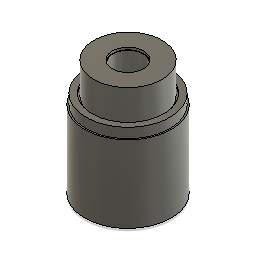
shaft (Autodesk Fusion 360 design; units mm, degrees)
Autodesk Fusion 360 part; units mm, degrees
note: some values were not read from the file. Chosen so that the rebuilt part matches the saved one: which face or edge a step refers to; where a thread starts. Set by a fixed rule: which sketch regions a step uses.
sketch "Sketch1" plane through (0, 0, 0) normal (0, 1, 0) x (1, 0, 0) in component "Eixo"
  circle A0 centre (0, 0) radius 7.5
  dimension "d1" = 15
  constraint coincident A0.centre origin
  measures "d1" diameter of A0
extrude "Extrude1" add sketch "Sketch1" along normal blind 25 in component "Eixo"
sketch "Sketch2" plane through (0, 25, 0) normal (0, 1, 0) x (-1, 0, 0) in component "Eixo"
  circle A0 centre (0, 0) radius 7.5
  circle A1 centre (0, 0) radius 5.9
  dimension "d4" = 11.8
  constraint concentric A0 A1
  measures "d4" diameter of A1
extrude "Extrude2" add sketch "Sketch2" along normal blind 5 contours A1 in component "Eixo"
sketch "Sketch3" plane through (0, 30, 0) normal (0, 1, 0) x (-1, 0, 0) in component "Eixo"
  circle A0 centre (0, 0) radius 5.9
  circle A1 centre (0, 0) radius 2.45
  dimension "d7" = 4.9
  constraint coincident A0.centre A1.centre
  measures "d7" diameter of A1
extrude "Extrude3" add sketch "Sketch3" along normal blind 16 contours A1 in component "Eixo"
sketch "Sketch5" plane through (0, 0, 0) normal (0, -1, 0) x (1, 0, 0) in component "Eixo"
  circle A0 centre (0, 0) radius 7.5
  circle A1 centre (0, 0) radius 3.965
  dimension "d13" = 7.93
  constraint coincident A0.centre A1.centre
  measures "d13" diameter of A1
extrude "Extrude5" cut sketch "Sketch5" against normal blind 20 contours A1 in component "Eixo"
thread "Thread2" "ANSI Unified Screw Threads 0.375 3/8-16 UNC 3B" major diameter 9.525 minor diameter 7.94 pitch 1.5875 angle 60 modelled right hand crest width 0.1984 on face at (3.9521, 13.3333, -0.319) crest through (3.97, -0.893, 0) in component "Eixo"
sketch "Sketch6" plane through (0, 25, 0) normal (0, 1, 0) x (-1, 0, 0) in component "Eixo"
  circle A0 centre (0, 0) radius 5.9
  circle A1 centre (0, 0) radius 7.5
  circle A2 centre (0, 0) radius 7.25
  circle A3 centre (0, 0) radius 6.2
  dimension "d16" = 14.5
  dimension "d17" = 12.4
  constraint coincident A0.centre A1.centre
  measures "d16" diameter of A2
  measures "d17" diameter of A3
extrude "Extrude6" cut sketch "Sketch6" against normal blind 0.2 contours A1 in component "Eixo"
sketch "Sketch7" plane through (0, 25, 0) normal (0, 1, 0) x (-1, 0, 0) in component "Eixo"
  circle A0 centre (0, 0) radius 7.25
  circle A1 centre (0, 0) radius 5.9
  circle A2 centre (0, 0) radius 6.2
  dimension "d20" = 12.4
  constraint coincident A0.centre A1.centre
  measures "d20" diameter of A2
extrude "Extrude7" cut sketch "Sketch7" against normal blind 0.4 contours A2 in component "Eixo"
sketch "Sketch8" plane through (0, 30, 0) normal (0, 1, 0) x (-1, 0, 0) in component "Eixo"
  circle A0 centre (0, 0) radius 2.45
  circle A1 centre (0, 0) radius 5.9
  circle A2 centre (0, 0) radius 2.7
  dimension "d23" = 5.4
  constraint coincident A0.centre A1.centre
  measures "d23" diameter of A2
extrude "Extrude8" cut sketch "Sketch8" against normal blind 0.4 contours A2 in component "Eixo"
sketch "Sketch1 (2)" plane through (0, 0, 0) normal (0, -1, 0) x (1, 0, 0)
  spline S0 degree 3 poles (1.1325, -4.6259) (0.5322, -4.7157) (-0.0797, -4.6894) (-1.2366, -4.4049) (-1.7725, -4.1576) (-2.6991, -3.4812) (-3.0858, -3.0652) (-3.6202, -2.1947) (-3.7952, -1.767) (-3.9926, -0.8864) (-4.0186, -0.4407) (-3.97, 0) knots 0 0 0 0 0.182097 0.182097 0.357707 0.357707 0.526827 0.526827 0.664894 0.664894 0.79837 0.79837 0.79837 0.79837
  arc A0 (-2.8072, 2.8072) -> (-3.97, 0) centre (0, 0) ccw
  spline S1 degree 3 poles (-2.8072, 2.8072) (-2.4792, 3.2165) (-2.073, 3.5564) (-1.1358, 4.0756) (-0.6098, 4.2428) (0.4983, 4.3727) (1.0705, 4.3259) (2.1003, 4.0381) (2.5558, 3.8234) (3.3925, 3.2469) (3.765, 2.885) (4.0718, 2.4702) knots 0 0 0 0 0.157342 0.157342 0.321158 0.321158 0.491446 0.491446 0.641085 0.641085 0.795325 0.795325 0.795325 0.795325
  arc A1 (1.1325, -4.6259) -> (4.0718, 2.4702) centre (0, 0) ccw
  circle A2 centre (0, 0) radius 7.5
  circle A3 centre (0, 0) radius 7.5
  constraint concentric A0 A3
extrude "Extrude9" cut sketch "Sketch1 (2)" against normal blind 10 contours S0 A0 S1 A1 | A2 A3 in component "Eixo"
sketch "Sketch2 (2)" plane through (0, 46, 0) normal (0, 1, 0) x (-1, 0, 0)
  circle A0 centre (0, 0) radius 2.45
  circle A1 centre (0, 0) radius 2.6
  dimension "d28" = 5.2
  constraint coincident A0.centre A1.centre
  measures "d28" diameter of A1
extrude "Extrude10" cut sketch "Sketch2 (2)" against normal up to surface (26 mm away) contours A0 | A1 in component "Eixo"
sketch "Sketch3 (2)" plane through (0, 20, 0) normal (0, -1, 0) x (1, 0, 0)
  circle A0 centre (0, 0) radius 2.6
  spline S0 degree 3 poles (3.2347, -2.3016) (3.5298, -1.9707) (3.7671, -1.5925) (4.1168, -0.7605) (4.2222, -0.3106) (4.2914, 0.7086) (4.2174, 1.2716) (3.8546, 2.36) (3.5614, 2.8722) (2.7836, 3.7747) (2.3003, 4.1508) (1.7591, 4.4257) knots -0.79837 -0.79837 -0.79837 -0.79837 -0.664894 -0.664894 -0.526827 -0.526827 -0.357707 -0.357707 -0.182097 -0.182097 0 0 0 0
  arc A1 (1.7591, 4.4257) -> (-4.7498, 0.348) centre (0, 0) ccw
  spline S1 degree 3 poles (-4.7498, 0.348) (-4.7402, -0.1679) (-4.6466, -0.6788) (-4.2991, -1.6335) (-4.0524, -2.0726) (-3.3802, -2.9041) (-2.941, -3.2739) (-1.9629, -3.8105) (-1.4374, -3.9793) (-0.3727, -4.0995) (0.1553, -4.0581) (0.6598, -3.9148) knots -0.795325 -0.795325 -0.795325 -0.795325 -0.641085 -0.641085 -0.491446 -0.491446 -0.321158 -0.321158 -0.157342 -0.157342 0 0 0 0
  arc A2 (0.6598, -3.9148) -> (3.2347, -2.3016) centre (0, 0) ccw
  circle A3 centre (0, 0) radius 2.6
  line L0 (0, 0) -> (-2, 0)
  line L1 (-2, 0) -> (-2, 2.7045)
  line L2 (-2, 2.7045) -> (-2, -2.5)
  constraint concentric A0 A3
  constraint coincident A0.centre A1.centre
  constraint horizontal L0
  constraint perpendicular L0 L1
  constraint parallel L1 L2
extrude "Extrude11" add sketch "Sketch3 (2)" against normal blind 4 contours A0 A3 L1 L2 picked at (-2.3917, -0.1198) in component "Eixo"
sketch "Sketch4" plane through (0, 24.8, 0) normal (0, 1, 0) x (-1, 0, 0)
  circle A0 centre (0, 0) radius 7.25
  circle A1 centre (0, 0) radius 7.5
  circle A2 centre (0, 0) radius 7.25
  dimension "d33" = 14.5
  constraint coincident A0.centre A1.centre
  measures "d33" diameter of A2
extrude "Extrude12" cut sketch "Sketch4" against normal blind 1.5 in component "Eixo"
sketch "Sketch4 (2)" plane through (0, 0, 0) normal (0, -1, 0) x (1, 0, 0) in component "Eixo"
  circle A0 centre (0, 0) radius 7.5
  circle A1 centre (0, 0) radius 4
  dimension "d10" = 8
  constraint coincident A0.centre A1.centre
  measures "d10" diameter of A1
extrude "Extrude4" [suppressed] in component "Eixo"
thread "Thread1" [suppressed] in component "Eixo"
component "Eixo" placed x (1, 0, 0) y (0, 1, 0) z (0, 0, 1) at (0, 0, 0)
